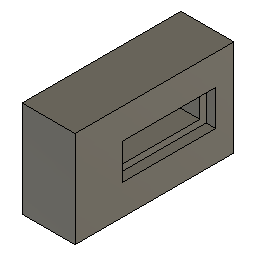
skadis_nut_coupon (Autodesk Fusion 360 design; units mm, degrees)
part number: 2026-09-06-14-40-16-018
Autodesk Fusion 360 part; units mm, degrees
sketch "Plate" plane through (0, 0, 0) normal (0, 1, 0) x (1, 0, 0)
  line L0 (0, 0) -> (11, 0)
  line L1 (11, 0) -> (11, -20)
  line L2 (11, -20) -> (0, -20)
  line L3 (0, -20) -> (0, 0)
  dimension "d23" = 11
  dimension "d24" = 20
  constraint coincident L0.start L3.end
  constraint horizontal L0
  constraint horizontal L2
  constraint vertical L1
  constraint vertical L3
  measures "d23" horizontal distance of L0.start L1.end
  measures "d24" vertical distance of L0.start L1.end
extrude "Plate (1)" add sketch "Plate" along normal mid plane 33 from surface at 4.5
sketch "Nut channel" plane through (0, 0, 0) normal (0, 1, 0) x (1, 0, 0)
  line L0 (9, -6.3) -> (12, -6.3)
  line L1 (12, -6.3) -> (12, -13.7)
  line L2 (12, -13.7) -> (9, -13.7)
  line L3 (9, -13.7) -> (9, -6.3)
  dimension "d28" = 12
  dimension "d29" = 6.3
  dimension "d30" = 3
  dimension "d31" = 7.4
  constraint horizontal L0
  constraint horizontal L2
  constraint vertical L1
  constraint vertical L3
  measures "d28" horizontal distance of origin L0.end
  measures "d29" vertical distance of origin L0.end
  measures "d30" horizontal distance of L0.start L0.end
  measures "d31" vertical distance of L0.end L1.end
extrude "Nut channel (1)" cut sketch "Nut channel" along normal mid plane 19.4 from surface at 7.52
sketch "Screw relief" plane through (0, 0, 0) normal (0, 1, 0) x (1, 0, 0)
  line L0 (-1, -7.6) -> (12, -7.6)
  line L1 (12, -7.6) -> (12, -12.4)
  line L2 (12, -12.4) -> (-1, -12.4)
  line L3 (-1, -12.4) -> (-1, -7.6)
  dimension "d35" = 12
  dimension "d36" = 7.6
  dimension "d37" = 13
  dimension "d38" = 4.8
  constraint horizontal L0
  constraint horizontal L2
  constraint vertical L1
  constraint vertical L3
  measures "d35" horizontal distance of origin L0.end
  measures "d36" vertical distance of origin L0.end
  measures "d37" horizontal distance of L0.start L0.end
  measures "d38" vertical distance of L0.end L1.end
extrude "Screw relief (1)" cut sketch "Screw relief" along normal mid plane 16.8 from surface at 7.52
equation "bracketWidth = 24.0 mm" comment "bracket width across the upright"
equation "plateHeight = 20.0 mm" comment "plate height"
equation "plateInboardExtension = 9.0 mm" comment "extra plate toward the desk centre, where the channel reaches"
equation "boardThickness = 6.0 mm" comment "measured SKADIS panel thickness"
equation "screwLength = 15.0 mm" comment "measured decorative M4 screw"
equation "screwDiameter = 4.0 mm" comment "M4 shank"
equation "screwClearance = 0.8 mm" comment "slack around the shank"
equation "screwTipClearance = 2.2 mm" comment "tip stops this short of the plate's back face"
equation "screwSlotWidth = screwDiameter + screwClearance" comment "screw relief slot height"
equation "nutAcrossFlats = 7.0 mm" comment "M4 square nut across flats"
equation "nutThickness = 2.2 mm" comment "M4 square nut thickness"
equation "nutChannelClearance = 0.4 mm" comment "slack around the nut in its channel"
equation "nutProud = 0.2 mm" comment "nut stands out of the pocket to be clamped"
equation "nutPocketDepth = nutThickness - nutProud" comment "channel depth"
equation "nutChannelHeight = nutAcrossFlats + nutChannelClearance" comment "channel height; under the nut's diagonal so it cannot turn"
equation "plateThickness = screwLength - boardThickness - nutProud + screwTipClearance" comment "derived: deep enough to swallow the screw"
equation "mountTravel = 12.0 mm" comment "left-right adjustment"
equation "nutChannelLength = mountTravel + nutAcrossFlats + nutChannelClearance" comment "channel length along the plate"
equation "screwSlotLength = mountTravel + screwSlotWidth" comment "relief slot length along the plate"
equation "topMountZ = 10.0 mm" comment "top channel centre"
equation "mountOffsetY = 7.52 mm" comment "channel centre on the board's grid"
equation "slotOvershoot = 1.0 mm" comment "cuts reach past the faces they cut"
equation "d23 = plateThickness"
equation "d24 = plateHeight"
equation "d25 = plateInboardExtension / 2"
equation "d26 = bracketWidth + plateInboardExtension"
equation "d28 = plateThickness + slotOvershoot"
equation "d29 = topMountZ - nutChannelHeight / 2"
equation "d30 = nutPocketDepth + slotOvershoot"
equation "d31 = nutChannelHeight"
equation "d32 = mountOffsetY"
equation "d33 = nutChannelLength"
equation "d35 = plateThickness + slotOvershoot"
equation "d36 = topMountZ - screwSlotWidth / 2"
equation "d37 = plateThickness + 2 * slotOvershoot"
equation "d38 = screwSlotWidth"
equation "d39 = mountOffsetY"
equation "d40 = screwSlotLength"
named bodies: "skadis_nut_coupon"
